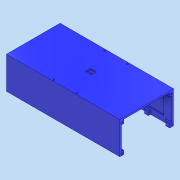
# Autodesk Inventor part: electronics_case
Saved by Autodesk Inventor 2022 (Build 260153000, 153)
## iProperties
Created: 2021-09-13
Part Number: electronics_case
Material: Generic
Document SubType Name: Modeling
Designer: nnico
Density: 1 g/cm^3
Appearance: Blue - Wall Paint - Glossy
Author: nnico
Autodesk Inventor part; units mm, degrees
ref_plane "YZ Plane" through (0, 0, 0) normal (1, 0, 0) x (0, 1, 0)
ref_plane "XZ Plane" through (0, 0, 0) normal (0, 1, 0) x (-1, 0, 0)
ref_plane "XY Plane" through (0, 0, 0) normal (0, 0, 1) x (1, 0, 0)
sketch "Sketch1" plane through (0, 0, 0) normal (0, 1, 0) x (-1, 0, 0)
  line L0 (146, -66) -> (-146, -66)
  line L1 (-146, -66) -> (-146, 66) construction
  line L2 (-146, 66) -> (146, 66)
  line L3 (146, 66) -> (146, -66)
  line L4 (146, 0) -> (-146, 0) construction
  line L5 (0, 66) -> (0, -66) construction
  line L6 (150, -70) -> (-146, -70)
  line L7 (-146, 70) -> (150, 70)
  line L8 (150, 70) -> (150, -70)
  line L9 (-146, 66) -> (-146, 70)
  line L10 (-146, -66) -> (-146, -70)
  point P0 (0, 0)
  point P1 (0, 0)
  dimension "d0" = 292
  dimension "d1" = 132
  dimension "d2" = 4
  dimension "d3" = 4
  constraints: 22 end point, 5 midpoint, 3 parallel, 2 horizontal, 2 perpendicular, 1 coincident, 1 point on line, 1 other
  measures "d0" distance of L0.start L0.end
  measures "d1" distance of L2.end L0.start
  measures "d2" distance between parallel lines of L8 L3
  measures "d3" distance of L6.end L0.end
extrude "Extrusion1" add sketch "Sketch1" along normal blind 80
sketch "Sketch2" plane through (0, 0, 0) normal (0, -1, 0) x (1, 0, 0)
  line L0 (146, 66) -> (-146, 66) construction
  line L1 (-146, -66) -> (146, -66) construction
  line L2 (146, 66) -> (146, -66) construction
  line L3 (146, 0) -> (-146, 0) construction
  line L4 (-146, 66) -> (-146, -66) construction
  line L5 (-90, 66) -> (-90, 60)
  line L6 (-90, 60) -> (-80, 60)
  line L7 (-80, 60) -> (-80, 66)
  line L8 (-90, -66) -> (-90, -60)
  line L9 (-90, -60) -> (-80, -60)
  line L10 (-80, -60) -> (-80, -66)
  line L11 (0, 66) -> (0, -66) construction
  line L12 (90, 66) -> (90, 60)
  line L13 (90, 60) -> (80, 60)
  line L14 (80, 60) -> (80, 66)
  line L15 (80, -60) -> (80, -66)
  line L16 (90, -60) -> (80, -60)
  line L17 (90, -66) -> (90, -60)
  line L18 (-90, 66) -> (-80, 66)
  line L19 (-80, -66) -> (-90, -66)
  line L20 (90, -66) -> (80, -66)
  line L21 (80, 66) -> (90, 66)
  point P0 (0, 0)
  dimension "d6" = 6
  dimension "d7" = 56
  dimension "d8" = 10
  constraints: 38 end point, 12 symmetric about line, 4 collinear, 4 midpoint, 2 perpendicular, 2 point on line, 1 horizontal, 1 vertical
  measures "d6" distance of L5.start L5.end
  measures "d7" distance of L0.end L5.start
  measures "d8" distance of L5.end L6.end
extrude "Extrusion2" add sketch "Sketch2" against normal blind 10
sketch "Sketch3" plane through (-150, 0, -70) normal (-1, 0, 0) x (0, 0, 1)
  line L0 (136, 10) -> (130, 10) construction
  line L1 (10, 10) -> (4, 10) construction
  line L2 (10, 10) -> (4, 10) construction
  line L3 (130, 10) -> (136, 10) construction
  line L4 (10, 10) -> (130, 10) construction
  line L5 (136, 80) -> (4, 80) construction
  line L6 (70, 80) -> (70, 0) construction
  line L7 (0, 0) -> (140, 0) construction
  line L8 (0, 0) -> (0, 80) construction
  line L9 (0, 14) -> (140, 14) construction
  circle A0 centre (36, 14) radius 1.5
  circle A1 centre (104, 14) radius 1.5
  line L10 (0, 0) -> (0, 80) construction
  line L11 (0, 46) -> (140, 46) construction
  line L12 (140, 0) -> (140, 80) construction
  circle A2 centre (36, 46) radius 1.5
  circle A3 centre (104, 46) radius 1.5
  dimension "d11" = 4
  dimension "d12" = 3
  dimension "d13" = 68
  dimension "d26" = 32
  dimension "d27" = 3
  constraints: 8 end point, 5 point on line, 4 centre point, 3 horizontal, 2 symmetric about line, 1 midpoint, 1 perpendicular, 2 other
  measures "d11" vertical distance of L9.end L0.end
  measures "d12" diameter of A0
  measures "d13" diameter of A0.centre L6
  measures "d26" distance of L11.start L9.start
  measures "d27" diameter of A2
extrude "Extrusion3" cut sketch "Sketch3" against normal blind 10
sketch "Sketch4" plane through (0, 0, 0) normal (0, -1, 0) x (1, 0, 0)
  line L0 (146, 66) -> (-146, 66) projected
  line L1 (146, 66) -> (136, 66)
  line L2 (136, 66) -> (136, 60)
  line L3 (136, 60) -> (146, 60)
  line L4 (146, 60) -> (146, 66)
  line L5 (146, -66) -> (146, -70) construction
  line L6 (146, -66) -> (146, 66) construction
  line L7 (146, 0) -> (-146, 0) construction
  line L8 (-146, 66) -> (-146, -66) construction
  line L9 (146, -66) -> (136, -66)
  line L10 (136, -66) -> (136, -60)
  line L11 (136, -60) -> (146, -60)
  line L12 (146, -60) -> (146, -66)
  point P0 (0, 0)
  dimension "d16" = 10
  dimension "d17" = 6
  constraints: 20 end point, 3 symmetric about line, 2 midpoint, 2 parallel, 1 horizontal, 1 perpendicular, 1 vertical
  measures "d16" distance of L3.end L2.end
  measures "d17" distance of L2.end L1.end
extrude "Extrusion4" add sketch "Sketch4" against normal blind 10
sketch "Sketch6" plane through (146, 0, 70) normal (1, 0, 0) x (0, 0, -1)
  line L0 (4, 0) -> (4, 80) construction
  line L1 (136, 10) -> (136, 80) construction
  line L2 (4, 80) -> (136, 80) construction
  line L3 (4, 0) -> (10, 0) construction
  line L4 (130, 0) -> (130, 10) construction
  line L5 (10, 0) -> (130, 0) construction
  line L6 (140, 80) -> (0, 80) construction
  line L7 (70, 80) -> (70, 0) construction
  line L8 (4, 80) -> (10, 80)
  line L9 (10, 80) -> (10, 70)
  line L10 (10, 70) -> (4, 70)
  line L11 (4, 70) -> (4, 80)
  line L12 (136, 0) -> (136, 80) construction
  line L13 (136, 80) -> (4, 80) construction
  line L14 (0, 80) -> (140, 80) construction
  line L15 (136, 80) -> (130, 80)
  line L16 (130, 80) -> (130, 70)
  line L17 (130, 70) -> (136, 70)
  line L18 (136, 70) -> (136, 80)
  dimension "d20" = 10
  constraints: 28 end point, 8 symmetric about line, 3 horizontal, 2 parallel, 1 midpoint, 1 perpendicular, 1 vertical
  measures "d20" distance of L8.end L9.end
extrude "Extrusion5" add sketch "Sketch6" against normal blind 10
sketch "Sketch7" plane through (146, 0, 70) normal (1, 0, 0) x (0, 0, -1)
  line L0 (0, 80) -> (10, 80) construction
  line L1 (10, 70) -> (4, 70) construction
  line L2 (0, 80) -> (10, 70) construction
  line L3 (10, 80) -> (0, 70) construction
  line L4 (0, 0) -> (0, 80) construction
  line L5 (0, 40) -> (140, 40) construction
  line L6 (140, 0) -> (140, 80) construction
  line L7 (70, 0) -> (70, 80) construction
  line L8 (140, 80) -> (0, 80) construction
  circle A0 centre (5, 75) radius 2.5
  circle A1 centre (135, 75) radius 2.5
  circle A2 centre (5, 5) radius 2.5
  circle A3 centre (135, 5) radius 2.5
  dimension "d23" = 5
  constraints: 8 end point, 4 centre point, 4 midpoint, 3 symmetric about line, 1 point on line, 3 other
  measures "d23" diameter of A0
extrude "Extrusion6" cut sketch "Sketch7" against normal blind 6
sketch "Sketch8" plane through (0, 80, 0) normal (0, 1, 0) x (1, 0, 0)
  line L0 (146, 70) -> (146, 60) projected
  line L1 (-150, 70) -> (-150, -70) projected
  line L2 (146, 70) -> (-150, 70)
  line L3 (-150, 70) -> (-150, -70)
  line L4 (-150, -70) -> (146, -70)
  line L5 (146, -70) -> (146, 70)
  point P0 (0, 0)
  constraints: 8 end point, 2 parallel, 1 horizontal, 1 perpendicular
extrude "Extrusion7" add sketch "Sketch8" along normal blind 4
sketch "Sketch11" plane through (0, 0, 0) normal (0, -1, 0) x (1, 0, 0)
  circle A0 centre (85, 65) radius 2.5
  line L0 (-150, 70) -> (146, 70) projected
  line L1 (90, 60) -> (90, 66) projected
  line L2 (80, 66) -> (-80, 66) projected
  line L3 (0, 66) -> (0, -66) construction
  line L4 (-80, -66) -> (80, -66) projected
  circle A1 centre (-85, 65) radius 2.5
  line L5 (146, 60) -> (136, 60) construction
  line L6 (146, 60) -> (146, -60) construction
  line L7 (146, 60) -> (146, -60) construction
  line L8 (146, 0) -> (-146, 0) construction
  line L9 (-146, 66) -> (-146, -66) construction
  circle A2 centre (85, -65) radius 2.5
  circle A3 centre (-85, -65) radius 2.5
  point P0 (0, 0)
  dimension "d39" = 5
  dimension "d40" = 5
  dimension "d41" = 5
  constraints: 6 end point, 4 centre point, 4 midpoint, 3 symmetric about line, 1 vertical, 3 other
  measures "d39" diameter of A0
  measures "d40" distance from line of L0 A0.centre
  measures "d41" distance from line of L1 A0.centre
extrude "Extrusion8" cut sketch "Sketch11" against normal blind 6
sketch "Sketch12" plane through (-90, 0, 60) normal (-1, 0, 0) x (0, 0, 1)
  line L0 (6, 0) -> (0, 0) projected
  line L1 (6, 10) -> (6, 0) projected
  line L2 (0, 10) -> (6, 10) projected
  line L3 (0, 0) -> (0, 10) projected
  line L4 (-120, 0) -> (-126, 0) projected
  line L5 (-120, 0) -> (-120, 10) projected
  line L6 (-126, 10) -> (-120, 10) projected
  line L7 (-126, 0) -> (-126, 10) projected
  point P0 (-60, 0)
  point P1 (10, 84)
extrude "Extrusion9" add sketch "Sketch12" along normal blind 6
sketch "Sketch13" plane through (80, 0, 60) normal (-1, 0, 0) x (0, 0, 1)
  line L0 (6, 0) -> (0, 0) projected
  line L1 (6, 10) -> (6, 0) projected
  line L2 (0, 10) -> (6, 10) projected
  line L3 (0, 0) -> (0, 10) projected
  line L4 (-120, 0) -> (-126, 0) projected
  line L5 (-120, 0) -> (-120, 10) projected
  line L6 (-126, 10) -> (-120, 10) projected
  line L7 (-126, 0) -> (-126, 10) projected
  point P0 (-60, 0)
extrude "Extrusion10" add sketch "Sketch13" along normal blind 6
sketch "Sketch14" plane through (136, 0, 60) normal (-1, 0, 0) x (0, 0, 1)
  line L0 (6, 0) -> (0, 0) projected
  line L1 (6, 10) -> (6, 0) projected
  line L2 (0, 10) -> (6, 10) projected
  line L3 (0, 0) -> (0, 10) projected
  line L4 (-120, 0) -> (-126, 0) projected
  line L5 (-120, 0) -> (-120, 10) projected
  line L6 (-126, 10) -> (-120, 10) projected
  line L7 (-126, 0) -> (-126, 10) projected
  line L8 (0, 70) -> (6, 70) projected
  line L9 (6, 80) -> (6, 70) projected
  line L10 (6, 80) -> (0, 80) projected
  line L11 (0, 80) -> (0, 70) projected
  line L12 (-120, 70) -> (-120, 80) projected
  line L13 (-120, 80) -> (-126, 80) projected
  line L14 (-126, 70) -> (-126, 80) projected
  line L15 (-126, 70) -> (-120, 70) projected
  point P0 (-60, 0)
extrude "Extrusion11" add sketch "Sketch14" along normal blind 6
chamfer "Chamfer4" distance 6 angle 45 8 edges at (130, 5, 60) (130, 5, -60) (130, 75, -60) (130, 75, 60) (74, 5, 60) (74, 5, -60) (-96, 5, 60) (-96, 5, -60)
sketch "Sketch16" plane through (0, 84, 0) normal (0, 1, 0) x (1, 0, 0)
  line L0 (-30, 66) -> (30, 66) construction
  line L1 (30, 66) -> (30, -66) construction
  line L2 (30, -66) -> (-30, -66) construction
  line L3 (-30, -66) -> (-30, 66) construction
  line L4 (146, 70) -> (-150, 70) construction
  line L5 (-150, -70) -> (146, -70) construction
  line L6 (-2, 70) -> (-2, -70) construction
  line L7 (-150, 70) -> (-150, -70) construction
  line L8 (-150, 0) -> (146, 0) construction
  line L9 (146, -60) -> (146, 60) construction
  line L10 (0, 66) -> (0, -66) construction
  line L11 (-30, 0) -> (30, 0) construction
  circle A0 centre (-30, 66) radius 1.75
  circle A1 centre (30, 66) radius 1.75
  circle A2 centre (-30, -66) radius 1.75
  circle A3 centre (30, -66) radius 1.75
  line L12 (7.5, -6.5) -> (-7.5, -6.5)
  line L13 (-7.5, -6.5) -> (-7.5, 6.5)
  line L14 (-7.5, 6.5) -> (7.5, 6.5)
  line L15 (7.5, 6.5) -> (7.5, -6.5)
  line L16 (7.5, 0) -> (-7.5, 0) construction
  line L17 (0, 6.5) -> (0, -6.5) construction
  point P0 (0, 0)
  point P1 (0, 0)
  dimension "d79" = 60
  dimension "d80" = 132
  dimension "d81" = 4
  dimension "d82" = 3.5
  dimension "d85" = 15
  dimension "d86" = 13
  constraints: 28 end point, 14 midpoint, 4 centre point, 4 parallel, 3 symmetric about line, 2 horizontal, 2 perpendicular, 1 coincident, 1 collinear, 3 other
  measures "d79" distance of L1.end L2.end
  measures "d80" distance of L0.end L1.end
  measures "d81" diameter of L6.end L10
  measures "d82" diameter of A0
  measures "d85" distance of L13.end L14.end
  measures "d86" distance of L12.end L13.end
extrude "Extrusion13" cut sketch "Sketch16" against normal blind 4
sketch "Sketch17" plane through (0, 80, 0) normal (0, -1, 0) x (1, 0, 0)
  line L0 (28.25, 66) -> (-28.25, 66) projected
  line L1 (-26, 66) -> (-38, 66)
  line L2 (-38, 66) -> (-38, 62)
  line L3 (-38, 62) -> (-26, 62)
  line L4 (-26, 62) -> (-26, 66)
  line L5 (0, 66) -> (0, -66) construction
  line L6 (-80, -66) -> (74, -66) construction
  line L7 (-146, 66) -> (-146, -66) construction
  line L8 (-146, 0) -> (146, 0) construction
  line L9 (146, 60) -> (146, -60) construction
  arc A0 (-31.75, 66) -> (-28.25, 66) centre (-30, 66) ccw construction
  line L10 (-30, 66) -> (-30, 62) construction
  line L11 (-28.25, 66) -> (28.25, 66)
  line L12 (28.25, -66) -> (-28.25, -66)
  line L13 (-26, -66) -> (-38, -66)
  line L14 (-38, -66) -> (-38, -62)
  line L15 (-38, -62) -> (-26, -62)
  line L16 (-26, -62) -> (-26, -66)
  arc A1 (-28.25, -66) -> (-31.75, -66) centre (-30, -66) ccw construction
  line L17 (-30, -66) -> (-30, -62) construction
  line L18 (-28.25, -66) -> (28.25, -66)
  line L19 (130, 66) -> (31.75, 66) projected
  line L20 (34, 66) -> (22, 66)
  line L21 (22, 66) -> (22, 62)
  line L22 (22, 62) -> (34, 62)
  line L23 (34, 62) -> (34, 66)
  line L24 (31.75, 66) -> (28.25, 66) construction
  line L25 (30, 66) -> (30, 62) construction
  line L26 (34, -66) -> (22, -66)
  line L27 (22, -66) -> (22, -62)
  line L28 (22, -62) -> (34, -62)
  line L29 (34, -62) -> (34, -66)
  line L30 (31.75, -66) -> (28.25, -66) construction
  line L31 (30, -66) -> (30, -62) construction
  point P0 (0, 0)
  point P1 (-28.25, 66)
  point P2 (31.75, 66)
  dimension "d87" = 4
  dimension "d88" = 4
  dimension "d89" = 8
  dimension "d92" = 12
  dimension "d93" = 4
  dimension "d94" = 4
  constraints: 52 end point, 22 symmetric about line, 8 point on line, 4 midpoint, 4 parallel, 4 perpendicular, 2 horizontal, 2 point on circle, 1 centre point, 1 vertical, 1 other
  measures "d87" distance of L3.end L1.start
  measures "d88" distance of L3.end L10.end
  measures "d89" distance of L2.end L10.end
  measures "d92" distance of L22.end L21.end
  measures "d93" distance of L21.end L20.end
  measures "d94" distance of L22.end L25.end
extrude "Extrusion14" add sketch "Sketch17" along normal blind 4
chamfer "Chamfer5" distance 4 angle 45 4 edges at (-38, 78, 62) (22, 78, 62) (-38, 78, -62) (22, 78, -62)
sketch "Sketch18" plane through (0, 80, 0) normal (0, -1, 0) x (1, 0, 0)
  line L0 (-146, 66) -> (-146, -66) construction
  line L1 (130, 66) -> (146, 66) construction
  line L2 (-146, -66) -> (146, -66) construction
  line L3 (146, -66) -> (146, 66) construction
  line L4 (146, 66) -> (-146, 66) construction
  line L5 (-146, 66) -> (-146, -66) construction
  line L6 (136, 61) -> (-140, 61)
  line L7 (-140, 61) -> (-140, -61)
  line L8 (-140, -61) -> (136, -61)
  line L9 (136, -61) -> (136, 61)
  line L10 (146, 60) -> (146, -60) construction
  line L11 (146, 0) -> (-146, 0) construction
  line L12 (22, 66) -> (-26, 66) construction
  line L13 (-2, 66) -> (-2, -66) construction
  line L14 (-26, -66) -> (22, -66) construction
  point P0 (0, 0)
  dimension "d98" = 5
  dimension "d99" = 10
  constraints: 20 end point, 4 midpoint, 4 parallel, 2 horizontal, 2 perpendicular, 2 other
  measures "d98" distance from line of L4 L6.start
  measures "d99" distance between parallel lines of L3 L9
extrude "Extrusion15" cut sketch "Sketch18" against normal blind 2
sketch "Sketch19" plane through (90, 0, 66) normal (0, 0, -1) x (-1, 0, 0)
  line L0 (-35, 15) -> (231, 15)
  line L1 (231, 15) -> (231, 71)
  line L2 (231, 71) -> (-35, 71)
  line L3 (-35, 71) -> (-35, 15)
  line L4 (-40, 10) -> (-40, 0) projected
  line L5 (236, 0) -> (236, 80) projected
  line L6 (170, 10) -> (186, 10) projected
  line L7 (68, 76) -> (56, 76) projected
  point P0 (90, 0)
  dimension "d102" = 5
  dimension "d103" = 5
  dimension "d104" = 5
  dimension "d105" = 5
  constraints: 8 end point, 2 parallel, 1 horizontal, 1 perpendicular
  measures "d102" distance from line of L4 L0.start
  measures "d103" distance between parallel lines of L1 L5
  measures "d104" distance between parallel lines of L6 L0
  measures "d105" distance between parallel lines of L2 L7
extrude "Extrusion16" cut sketch "Sketch19" against normal blind 2
sketch "Sketch20" plane through (-80, 0, -66) normal (0, 0, 1) x (1, 0, 0)
  line L0 (-61, 71) -> (-61, 15) projected
  line L1 (205, 71) -> (-61, 71) projected
  line L2 (205, 15) -> (205, 71) projected
  line L3 (-61, 15) -> (205, 15) projected
  point P0 (80, 0)
extrude "Extrusion18" cut sketch "Sketch20" against normal blind 2
body "Solid1"
